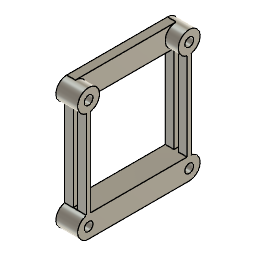
version_1 (Autodesk Fusion 360 design; units mm, degrees)
part number: 2025-10-18-19-38-59-563
Autodesk Fusion 360 part; units mm, degrees
sketch "Sketch6" plane through (0, 0, 0) normal (0, 1, 0) x (1, 0, 0)
  line L0 (-2, -80) -> (3, -80)
  line L1 (3, -80) -> (3, -57)
  line L2 (3, -57) -> (-2, -57)
  line L3 (-2, -57) -> (-2, -80)
  line L4 (-2, -58.5) -> (0, -58.5)
  line L5 (0, -58.5) -> (-0.3475, -58.5)
  line L6 (1, -58.5) -> (3, -58.5)
  line L7 (1, -58.5) -> (0, -58.5)
  line L8 (0, -58.5) -> (0, -78.5)
  line L9 (0, -78.5) -> (1, -78.5)
  line L10 (1, -78.5) -> (1, -58.5)
  line L11 (0, -78.5) -> (-2, -78.5)
  line L12 (1, -78.5) -> (3, -78.5)
  line L13 (0.5, -78.5) -> (0.5, -80)
  line L14 (0.5, -58.5) -> (0.5, -57)
  dimension "d51" = 5
  dimension "d52" = 23
  dimension "d53" = 2
  dimension "d54" = 2
  dimension "d55" = 20
  dimension "d56" = 2
  dimension "d57" = 2
  dimension "d58" = 1.5
  dimension "d59" = 1.5
  constraint horizontal L0
  constraint vertical L1
  constraint horizontal L2
  constraint vertical L3
  constraint coincident L3 L4.start
  constraint perpendicular L3 L4
  constraint coincident L1 L6.end
  constraint perpendicular L1 L6
  constraint horizontal L7
  constraint vertical L8
  constraint horizontal L9
  constraint vertical L10
  constraint coincident L3 L11.end
  constraint perpendicular L3 L11
  constraint coincident L1 L12.end
  constraint perpendicular L1 L12
  constraint midpoint L9 L13.start
  constraint midpoint L0 L13.end
  constraint vertical L14
  measures "d51" distance of L1.end L2.end
  measures "d52" distance of L0.end L1.end
  measures "d53" distance of L4.start L4.end
  measures "d54" distance of L6.start L6.end
  measures "d55" distance of L6.start L9.end
  measures "d56" distance of L8.end L11.end
  measures "d57" distance of L9.end L12.end
  measures "d58" distance of L13.start L13.end
  measures "d59" distance of L14.start L14.end
extrude "Extrude4" add sketch "Sketch6" along normal blind 1 contours L0 L3 L9 L11 L13 | L0 L1 L9 L12 L13 | L3 L4 L5 L8 L11 | L2 L3 L4 L5 L7 L14 | L1 L6 L10 L12 | L1 L2 L6 L7 L14 makes body 1
copy_body "CopyPasteBodies1" bodies 1 makes body 2
move_body "Move1" bodies 2 to x (1, 0, 0) y (0, 1, 0) z (0, 0, 1) at (0, 23, 0)
sketch "Sketch7" plane through (0, 0, 0) normal (1, 0, 0) x (0, 1, 0)
  line L0 (0.5, 78.5) -> (0.5, 79.5)
  line L1 (0.5, 79.5) -> (0.5, 81)
  circle A0 centre (0.5, 81) radius 1
  circle A1 centre (0.5, 81) radius 2.5
  line L2 (0.5, 58) -> (0.5, 56.5)
  line L3 (0.5, 57) -> (0.5, 56)
  circle A2 centre (0.5, 56) radius 1
  circle A3 centre (0.5, 56) radius 2.5
  line L4 (23.5, 58.5) -> (23.5, 57.5)
  line L5 (23.5, 57.5) -> (23.5, 56)
  circle A4 centre (23.5, 56) radius 1
  circle A5 centre (23.5, 56) radius 2.5
  line L6 (23.5, 78.5) -> (23.5, 79.5)
  line L7 (23.5, 79.5) -> (23.5, 81)
  circle A6 centre (23.5, 81) radius 1
  circle A7 centre (23.5, 81) radius 2.5
  dimension "d62" = 1
  dimension "d63" = 2
  dimension "d64" = 1.5
  dimension "d65" = 5
  dimension "d66" = 1.5
  dimension "d67" = 0.5
  dimension "d68" = 2
  dimension "d69" = 5
  dimension "d70" = 1
  dimension "d71" = 1.5
  dimension "d72" = 2
  dimension "d73" = 5
  dimension "d74" = 1
  dimension "d75" = 1.5
  dimension "d76" = 2
  dimension "d77" = 5
  constraint vertical L0
  constraint parallel L0 L1
  constraint coincident L1.end A0.centre
  constraint vertical L2
  constraint vertical L3
  constraint coincident L3.end A2.centre
  constraint coincident L3.start A2
  constraint concentric A2 A3
  constraint vertical L4
  constraint parallel L4 L5
  constraint coincident L5.end A4.centre
  constraint vertical L6
  constraint parallel L6 L7
  constraint coincident L7.end A6.centre
  constraint concentric A6 A7
  measures "d62" distance of L0.start L0.end
  measures "d63" diameter of A0
  measures "d64" distance of L0.end L1.end
  measures "d65" diameter of A1
  measures "d66" distance of L2.start L2.end
  measures "d67" distance of L2.end L3.end
  measures "d68" diameter of A2
  measures "d69" diameter of A3
  measures "d70" distance of L4.start L4.end
  measures "d71" distance of L4.end L5.end
  measures "d72" diameter of A4
  measures "d73" diameter of A5
  measures "d74" distance of L6.start L6.end
  measures "d75" distance of L6.end L7.end
  measures "d76" diameter of A6
  measures "d77" diameter of A7
extrude "Extrude5" add sketch "Sketch7" along normal blind 3 bodies 1 2
extrude "Extrude6" add 4 faces at (0, 22.4974, 57.1469) (0, -0.5026, 57.1469) (0, 25.015, 79.7012) (0, 2.015, 79.7012) along direction (-1, 0, 0) blind 2 on bodies 1 2 bodies 2 1
sketch "Sketch8" plane through (0, 0, 0) normal (1, 0, 0) x (0, 1, 0)
  line L0 (3, 81) -> (21, 81)
  line L1 (0.4686, 78.5) -> (23.5, 78.5)
  line L2 (0.4686, 78.5) -> (0.4686, 83.5)
  line L3 (23.5, 83.5) -> (23.5, 78.5)
  line L4 (0.4686, 83.5) -> (23.5, 83.5)
  line L5 (23.5, 83.5) -> (23.5, 78.5)
  line L6 (23.5, 78.5) -> (0.4686, 78.5)
  line L7 (0.4686, 78.5) -> (0.4686, 83.5)
  line L8 (0.4686, 82.0062) -> (1.4686, 82.0062)
  line L9 (1.4686, 82.0062) -> (1.4686, 80.0062)
  line L10 (1.4686, 80.0062) -> (0.4686, 80.0062)
  line L11 (1.4686, 82.0062) -> (23.5, 82.0062)
  line L12 (0.4686, 80.0062) -> (23.5, 80.0062)
  line L13 (22.4687, 82.0062) -> (22.4687, 80.0062)
  line L14 (0.5, 56) -> (23.5, 56)
  line L15 (23.5, 56) -> (23.5, 53.5)
  line L16 (23.5, 53.5) -> (0.5, 53.5)
  line L17 (0.5, 53.5) -> (0.5, 56)
  line L18 (0.5, 58.5) -> (23.5, 58.5)
  line L19 (23.5, 58.5) -> (23.5, 56)
  line L20 (0.5, 56) -> (0.5, 58.5)
  line L21 (1.5, 56) -> (1.5, 57)
  line L22 (1.5, 56) -> (1.5, 55)
  line L23 (1.5, 55) -> (0.5, 55)
  line L24 (1.5, 57) -> (0.5, 57)
  line L25 (23.5, 57) -> (22.5, 57)
  line L26 (22.5, 56) -> (22.5, 57)
  line L27 (22.5, 56) -> (22.5, 55)
  line L28 (22.5, 55) -> (23.5, 55)
  dimension "d82" = 2
  dimension "d83" = 1
  dimension "d84" = 2
  constraint horizontal L0
  constraint horizontal L1
  constraint vertical L2
  constraint perpendicular L1 L3
  constraint horizontal L4
  constraint vertical L5
  constraint horizontal L6
  constraint vertical L7
  constraint coincident L2 L8.start
  constraint perpendicular L2 L8
  constraint perpendicular L8 L9
  constraint coincident L7 L10.end
  constraint perpendicular L7 L10
  constraint coincident L3 L11.end
  constraint perpendicular L3 L11
  constraint coincident L5 L12.end
  constraint perpendicular L5 L12
  constraint coincident L11 L13.start
  constraint coincident L12 L13.end
  constraint perpendicular L12 L13
  constraint horizontal L14
  constraint perpendicular L14 L15
  constraint perpendicular L15 L16
  constraint perpendicular L14 L17
  constraint perpendicular L15 L18
  constraint perpendicular L14 L19
  constraint perpendicular L18 L20
  constraint coincident L14 L21.start
  constraint perpendicular L14 L21
  constraint perpendicular L14 L22
  constraint coincident L17 L23.end
  constraint perpendicular L17 L23
  constraint coincident L20 L24.end
  constraint perpendicular L20 L24
  constraint coincident L19 L25.start
  constraint perpendicular L19 L25
  constraint coincident L14 L26.start
  constraint perpendicular L14 L27
  constraint coincident L15 L28.end
  constraint perpendicular L15 L28
  measures "d82" distance of L8.end L9.end
  measures "d83" distance of L8.start L8.end
  measures "d84" distance of L11.end L12.end
extrude "Extrude7" add sketch "Sketch8" against normal blind 2 contours L1 L2 L3 L5 L6 L7 L10 L12 | L2 L3 L4 L5 L7 L8 L11 | L9 L11 L12 L13 bodies 1 2
extrude "Extrude8" add sketch "Sketch8" along normal blind 3 contours L14 L18 L19 L20 L21 L24 L25 L26 | L14 L15 L16 L17 L22 L23 L27 L28 bodies 1
extrude "Extrude9" add sketch "Sketch8" against normal blind 2 contours L14 L18 L19 L20 L21 L24 L25 L26 | L14 L15 L16 L17 L22 L23 L27 L28 bodies 1
